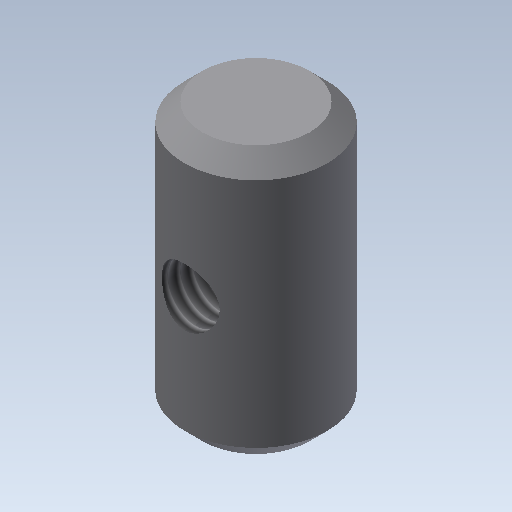
# Autodesk Inventor part: LANGMUTTER
Saved by Autodesk Inventor 2020.2 (Build 242310000, 310)
## iProperties
Created: 2014-02-21
Part Number: LANGMUTTER
Material: Allgemein
Document SubType Name: Modeling
Designer: g.schardt
Density: 1 g/cm^3
Appearance: Vorgabe
Mass: 0.666198 g
Surface Area: 5.06502 cm^2
Volume: 0.666198 cm^3
Author: g.schardt
Autodesk Inventor part; units mm, degrees
ref_plane "YZ Plane" through (0, 0, 0) normal (1, 0, 0) x (0, 1, 0)
ref_plane "XZ Plane" through (0, 0, 0) normal (0, 1, 0) x (-1, 0, 0)
sketch "Skizze1" plane through (0, 0, 0) normal (0, 0, 1) x (1, 0, 0)
  circle A0 centre (0, 0) radius 4
  point P0 (0, 4)
  dimension "d0" = 8
  constraints: 1 coincident, 1 vertical alignment, 2 other
extrude "Extrusion1" add sketch "Skizze1" along normal blind 15
ref_plane "Arbeitsebene1" through (0, 4, 0) normal (0, 1, 0) x (-1, 0, 0)
sketch "Skizze2" plane through (0, 4, 0) normal (0, 1, 0) x (-1, 0, 0)
  point P0 (0, 0)
  point P1 (0, 7.5)
  dimension "d3" = 7.5
  measures "d3" distance of point (0, 7.5) point (0, 0)
hole "Bohrung1" at (0, 4, 7.5) direction (0, -1, 0) diameter 3.242 end through all thread size "M4x0.7" class "6H" standard "ANSI Metric M Profile"
chamfer "Fase1" distance 1 angle 45 2 edges at (-4, 0, 0) (-4, 0, 15)
